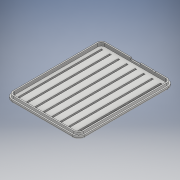
# Autodesk Inventor part: CaseGroboyBack
Saved by Autodesk Inventor 2017 SP1 (Build 210196100, 196)
## iProperties
Created: 2017-08-23
Part Number: CaseGroboyBack
Material: Generic
Document SubType Name: Modeling
Designer: Groguard
Density: 1 g/cm^3
Appearance: Default
Author: Groguard
Autodesk Inventor part; units mm, degrees
ref_plane "YZ Plane" through (0, 0, 0) normal (1, 0, 0) x (0, 1, 0)
ref_plane "XZ Plane" through (0, 0, 0) normal (0, 1, 0) x (-1, 0, 0)
ref_plane "XY Plane" through (0, 0, 0) normal (0, 0, 1) x (1, 0, 0)
sketch "Sketch6" plane through (0, 0, 0) normal (0, 0, 1) x (1, 0, 0)
  arc A0 (83, 106.5858) -> (78.5858, 111) centre (78.5858, 106.5858) ccw
  line L0 (83, 106.5858) -> (83, 3.4142)
  arc A1 (78.5858, -1) -> (83, 3.4142) centre (78.5858, 3.4142) ccw
  line L1 (78.5858, -1) -> (3.4142, -1)
  arc A2 (-1, 3.4142) -> (3.4142, -1) centre (3.4142, 3.4142) ccw
  line L2 (-1, 3.4142) -> (-1, 106.5858)
  arc A3 (3.4142, 111) -> (-1, 106.5858) centre (3.4142, 106.5858) ccw
  line L3 (3.4142, 111) -> (78.5858, 111)
  arc A4 (86, 106.5858) -> (78.5858, 114) centre (78.5858, 106.5858) ccw
  line L4 (86, 106.5858) -> (86, 3.4142)
  arc A5 (78.5858, -4) -> (86, 3.4142) centre (78.5858, 3.4142) ccw
  line L5 (78.5858, -4) -> (3.4142, -4)
  arc A6 (-4, 3.4142) -> (3.4142, -4) centre (3.4142, 3.4142) ccw
  line L6 (-4, 3.4142) -> (-4, 106.5858)
  arc A7 (3.4142, 114) -> (-4, 106.5858) centre (3.4142, 106.5858) ccw
  line L7 (3.4142, 114) -> (78.5858, 114)
  constraints: 16 end point, 16 point on circle, 8 centre point
extrude "Extrusion4" add sketch "Sketch6" along normal blind 3 contours L0 A1 L1 A2 L2 A3 L3 A0 | L4 A5 L5 A6 L6 A7 L7 A4
sketch "Sketch7" plane through (0, 0, 3) normal (0, 0, 1) x (1, 0, 0)
  line L0 (83, 106.5858) -> (83, 3.4142)
  line L1 (-1, 3.4142) -> (-1, 106.5858)
  arc A0 (78.5858, -1) -> (83, 3.4142) centre (78.5858, 3.4142) ccw
  arc A1 (-1, 3.4142) -> (3.4142, -1) centre (3.4142, 3.4142) ccw
  line L2 (78.5858, -1) -> (3.4142, -1)
  line L3 (3.4142, 111) -> (78.5858, 111)
  arc A2 (3.4142, 111) -> (-1, 106.5858) centre (3.4142, 106.5858) ccw
  arc A3 (83, 106.5858) -> (78.5858, 111) centre (78.5858, 106.5858) ccw
  line L4 (-4, 106.5858) -> (-4, 3.4142)
  arc A4 (-4, 3.4142) -> (3.4142, -4) centre (3.4142, 3.4142) ccw
  line L5 (3.4142, -4) -> (78.5858, -4)
  arc A5 (78.5858, -4) -> (86, 3.4142) centre (78.5858, 3.4142) ccw
  line L6 (86, 3.4142) -> (86, 106.5858)
  arc A6 (86, 106.5858) -> (78.5858, 114) centre (78.5858, 106.5858) ccw
  line L7 (78.5858, 114) -> (3.4142, 114)
  arc A7 (3.4142, 114) -> (-4, 106.5858) centre (3.4142, 106.5858) ccw
  point P0 (0, 0)
  dimension "d17" = 3
  constraints: 16 end point, 16 point on circle, 8 centre point, 7 other
  measures "d17" radial gap between concentric circles of A2 A7
extrude "Extrusion5" add sketch "Sketch7" along normal blind 4
sketch "Sketch8" plane through (0, 0, 7) normal (0, 0, 1) x (1, 0, 0)
  arc A0 (3.4142, 111) -> (-1, 106.5858) centre (3.4142, 106.5858) ccw
  line L0 (3.4142, 111) -> (78.5858, 111)
  arc A1 (83, 106.5858) -> (78.5858, 111) centre (78.5858, 106.5858) ccw
  line L1 (-1, 3.4142) -> (-1, 106.5858)
  line L2 (83, 106.5858) -> (83, 3.4142)
  arc A2 (-1, 3.4142) -> (3.4142, -1) centre (3.4142, 3.4142) ccw
  line L3 (78.5858, -1) -> (3.4142, -1)
  arc A3 (78.5858, -1) -> (83, 3.4142) centre (78.5858, 3.4142) ccw
  line L4 (-4, 106.5858) -> (-4, 3.4142)
  arc A4 (-4, 3.4142) -> (3.4142, -4) centre (3.4142, 3.4142) ccw
  line L5 (3.4142, -4) -> (78.5858, -4)
  arc A5 (78.5858, -4) -> (86, 3.4142) centre (78.5858, 3.4142) ccw
  line L6 (86, 3.4142) -> (86, 106.5858)
  arc A6 (86, 106.5858) -> (78.5858, 114) centre (78.5858, 106.5858) ccw
  line L7 (78.5858, 114) -> (3.4142, 114)
  arc A7 (3.4142, 114) -> (-4, 106.5858) centre (3.4142, 106.5858) ccw
  line L8 (-2.5, 106.5858) -> (-2.5, 3.4142)
  arc A8 (-2.5, 3.4142) -> (3.4142, -2.5) centre (3.4142, 3.4142) ccw
  line L9 (3.4142, -2.5) -> (78.5858, -2.5)
  arc A9 (78.5858, -2.5) -> (84.5, 3.4142) centre (78.5858, 3.4142) ccw
  line L10 (84.5, 3.4142) -> (84.5, 106.5858)
  arc A10 (84.5, 106.5858) -> (78.5858, 112.5) centre (78.5858, 106.5858) ccw
  line L11 (78.5858, 112.5) -> (3.4142, 112.5)
  arc A11 (3.4142, 112.5) -> (-2.5, 106.5858) centre (3.4142, 106.5858) ccw
  point P0 (0, 0)
  point P1 (0, 0)
  dimension "d20" = 3
  dimension "d21" = 1.5
  constraints: 24 end point, 24 point on circle, 12 centre point, 14 other
  measures "d20" radial gap between concentric circles of A0 A7
  measures "d21" radial gap between concentric circles of A7 A11
extrude "Extrusion6" cut sketch "Sketch8" against normal blind 3 contours A7 L7 A6 L6 A5 L5 A4 L4
fillet "Fillet2" radius 2 8 edges at (-1.8284, 111.8284, 0) (-4, 55, 0) (-1.8284, -1.8284, 0) (41, -4, 0) (83.8284, -1.8284, 0) (86, 55, 0) (83.8284, 111.8284, 0) (41, 114, 0)
sketch "Sketch9" plane through (3.4142, 111, 3) normal (0, -1, 0) x (1, 0, 0)
  circle A0 centre (60.4216, 6.636) radius 3.25
  line L0 (31.5858, 6) -> (43.5858, 6)
  line L1 (43.5858, 6) -> (43.5858, 2)
  line L2 (43.5858, 2) -> (31.5858, 2)
  line L3 (31.5858, 2) -> (31.5858, 6)
  line L4 (31.5858, 6) -> (43.5858, 2) construction
  line L5 (43.5858, 6) -> (31.5858, 2) construction
  point P0 (37.5858, 4)
  dimension "d55" = 12
  dimension "d56" = 4
  constraints: 12 end point, 2 midpoint, 2 parallel, 1 centre point, 1 horizontal, 1 perpendicular
  measures "d55" distance of L1.end L2.end
  measures "d56" distance of L0.end L1.end
extrude "Extrusion7" cut sketch "Sketch9" against normal blind 3
sketch "Sketch11" plane through (0, 0, 3) normal (0, 0, 1) x (1, 0, 0)
  line L0 (3.4142, 3.4142) -> (5.4142, 3.4142)
  line L1 (5.4142, 3.4142) -> (5.4142, 106.5858)
  line L2 (5.4142, 106.5858) -> (3.4142, 106.5858)
  line L3 (3.4142, 106.5858) -> (3.4142, 3.4142)
  line L4 (13.8642, 3.4142) -> (15.8642, 3.4142)
  line L5 (15.8642, 3.4142) -> (15.8642, 106.5858)
  line L6 (15.8642, 106.5858) -> (13.8642, 106.5858)
  line L7 (13.8642, 106.5858) -> (13.8642, 3.4142)
  line L8 (24.3142, 3.4142) -> (26.3142, 3.4142)
  line L9 (26.3142, 3.4142) -> (26.3142, 106.5858)
  line L10 (26.3142, 106.5858) -> (24.3142, 106.5858)
  line L11 (24.3142, 106.5858) -> (24.3142, 3.4142)
  line L12 (34.7642, 3.4142) -> (36.7642, 3.4142)
  line L13 (36.7642, 3.4142) -> (36.7642, 106.5858)
  line L14 (36.7642, 106.5858) -> (34.7642, 106.5858)
  line L15 (34.7642, 106.5858) -> (34.7642, 3.4142)
  line L16 (45.2142, 3.4142) -> (47.2142, 3.4142)
  line L17 (47.2142, 3.4142) -> (47.2142, 106.5858)
  line L18 (47.2142, 106.5858) -> (45.2142, 106.5858)
  line L19 (45.2142, 106.5858) -> (45.2142, 3.4142)
  line L20 (55.6642, 3.4142) -> (57.6642, 3.4142)
  line L21 (57.6642, 3.4142) -> (57.6642, 106.5858)
  line L22 (57.6642, 106.5858) -> (55.6642, 106.5858)
  line L23 (55.6642, 106.5858) -> (55.6642, 3.4142)
  line L24 (66.1142, 3.4142) -> (68.1142, 3.4142)
  line L25 (68.1142, 3.4142) -> (68.1142, 106.5858)
  line L26 (68.1142, 106.5858) -> (66.1142, 106.5858)
  line L27 (66.1142, 106.5858) -> (66.1142, 3.4142)
  line L28 (76.5642, 3.4142) -> (78.5642, 3.4142)
  line L29 (78.5642, 3.4142) -> (78.5642, 106.5858)
  line L30 (78.5642, 106.5858) -> (76.5642, 106.5858)
  line L31 (76.5642, 106.5858) -> (76.5642, 3.4142)
  dimension "d57" = 2
  dimension "d60" = 10.45
  constraints: 64 end point, 2 horizontal, 2 parallel, 1 collinear, 1 perpendicular, 55 other
  measures "d57" distance of L2.end L1.end
  measures "d60" distance of L1.end L5.end
extrude "Extrusion9" cut sketch "Sketch11" against normal blind 3
body "Solid2"
